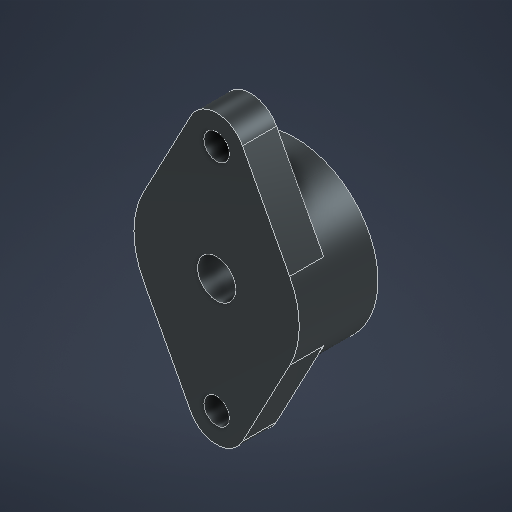
# Autodesk Inventor part: bearing_unit_15mm
Saved by Autodesk Inventor 2026 (Build 300175000, 175)
## iProperties
Created: 2026-05-04
Part Number: bearing_unit_15mm
Material: Чугун, серый
Document SubType Name: Modeling
Designer: user
Density: 7.15 g/cm^3
Appearance: Чугун серый
Mass: 824.689 g
Surface Area: 185.073 cm^2
Volume: 115.341 cm^3
Author: user
Autodesk Inventor part; units mm, degrees
ref_plane "YZ Plane" through (0, 0, 0) normal (1, 0, 0) x (0, 1, 0)
ref_plane "XZ Plane" through (0, 0, 0) normal (0, 1, 0) x (-1, 0, 0)
ref_plane "XY Plane" through (0, 0, 0) normal (0, 0, 1) x (1, 0, 0)
sketch "Эскиз1" plane through (0, 0, 0) normal (0, 0, 1) x (1, 0, 0)
  circle A0 centre (0, 0) radius 7.5
  circle A1 centre (0, 45) radius 5
  line L0 (46.4621, 0) -> (-49.3756, 0)
  arc A2 (10.171, 50.3667) -> (-10.171, 50.3667) centre (0, 45) ccw
  line L1 (-10.171, 50.3667) -> (-28.7441, 15.1667)
  line L2 (28.7441, 15.1667) -> (10.171, 50.3667)
  circle A3 centre (0, -45) radius 5
  arc A4 (-10.171, -50.3667) -> (10.171, -50.3667) centre (0, -45) ccw
  line L3 (-10.171, -50.3667) -> (-28.7441, -15.1667)
  line L4 (28.7441, -15.1667) -> (10.171, -50.3667)
  arc A5 (-28.7441, 15.1667) -> (-28.7441, -15.1667) centre (0, 0) ccw
  arc A6 (28.7441, -15.1667) -> (28.7441, 15.1667) centre (0, 0) ccw
  dimension "d0" = 15
  dimension "d2" = 10
  dimension "d4" = 45
  dimension "d5" = 23
  dimension "d6" = 32.5
  constraints: 10 end point, 8 point on circle, 7 centre point, 6 symmetric about line, 4 coincident, 4 tangent, 1 concentric, 1 horizontal, 1 vertical alignment, 2 other
  measures "d0" diameter of A0
  measures "d2" diameter of A1
  measures "d4" distance of A1.centre point (0, 0)
  measures "d5" diameter of A2
  measures "d6" radius of A6
extrude "Выдавливание1" add sketch "Эскиз1" along normal blind 13.4 contours L0 A6 L4 A4 L3 A5 A0 | A0 L0 A5 L1 A2 L2 A6
sketch "Эскиз2" plane through (0, 0, 0) normal (0, 0, -1) x (-1, 0, 0)
  circle A0 centre (0, 0) radius 7.5 projected
  line L0 (10.171, 50.3667) -> (28.7441, 15.1667) projected
  circle A1 centre (0, 0) radius 32.5
  constraints: 1 coincident, 3 other
extrude "Выдавливание2" add sketch "Эскиз2" along normal blind 17.6
